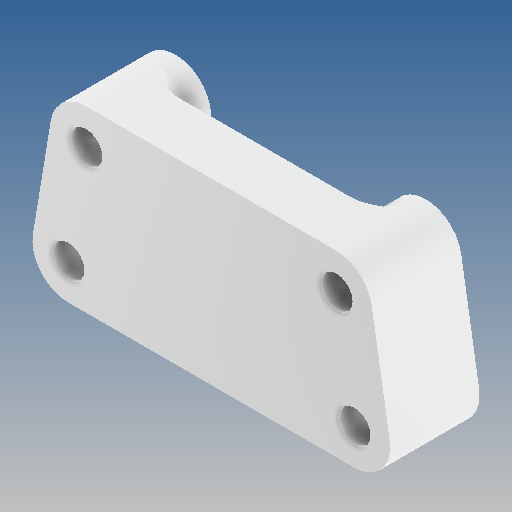
# Autodesk Inventor part: PWTR-0083
Saved by Autodesk Inventor 2021.1 (Build 251245000, 245)
## iProperties
Created: 2020-08-28
Part Number: PWTR-0083
Material: Aluminum 6061
Document SubType Name: Modeling
Designer: alid
Density: 2.7 g/cm^3
Appearance: Aluminum - Flat
Description: Handle Transfer Case Plate
Author: alid
Revision Number: A
Autodesk Inventor part; units mm, degrees
ref_plane "YZ Plane" through (0, 0, 0) normal (1, 0, 0) x (0, 1, 0)
ref_plane "XZ Plane" through (0, 0, 0) normal (0, 1, 0) x (-1, 0, 0)
ref_plane "XY Plane" through (0, 0, 0) normal (0, 0, 1) x (1, 0, 0)
sketch "Sketch1" plane through (0, 0, 0) normal (0, 1, 0) x (-1, 0, 0)
  line L0 (-40, -25) -> (40, -25)
  line L1 (35, 25) -> (-35, 25)
  line L2 (-49.863939, -13.35601) -> (-44.863939, 16.64399)
  line L3 (44.863939, 16.64399) -> (49.863939, -13.35601)
  circle A0 centre (-35, 15) radius 10
  circle A1 centre (-40, -15) radius 10
  circle A2 centre (35, 15) radius 10
  circle A3 centre (40, -15) radius 10
  line L4 (-35, 5) -> (35, 5)
  line L5 (-40, -5) -> (40, -5)
  line L6 (30.136061, -16.64399) -> (25.136061, 13.35601)
  line L7 (-25.136061, 13.35601) -> (-30.136061, -16.64399)
  point P0 (0, 0)
  point P1 (51.804604, -25)
  point P2 (0, 25)
  point P3 (0, -25)
  point P4 (0, -25)
  point P5 (-44.863939, 16.64399)
  dimension "d22" = 70
  dimension "d23" = 50
  dimension "d24" = 25
  dimension "d25" = 80
  dimension "d26" = 20
  constraints: 16 end point, 16 tangent, 15 point on circle, 4 centre point, 3 coincident, 3 equal radius, 3 midpoint, 3 vertical alignment, 2 point on line, 1 equal length, 1 horizontal, 1 parallel
  measures "d22" distance of L1.start L1.end
  measures "d23" distance between parallel lines of L0 L1
  measures "d24" distance from line of L0 point (0, 0)
  measures "d25" distance of L0.start L0.end
  measures "d26" diameter of A0
extrude "Extrusion1" add sketch "Sketch1" along normal blind 15
extrude "Extrusion2" add sketch "Sketch1" along normal blind 25 contours A1 | A3 | L2 A0 L4 L7 L5 A1 | A1 L5 L7 | L6 L5 A3 | A0 | L5 L6 L4 A2 L3 A3 | A0 L7 L4 | L6 A2 L4 | A2
fillet "Fillet1" radius 5 6 edges at (-27.6361, 15, -1.644) (-27.3698, 15, 21.4637) (-33.5363, 15, -22.6302) (27.6361, 15, -1.644) (33.5363, 15, -22.6302) (27.3698, 15, 21.4637)
hole "Hole2" at (-35, 0, 15) direction (0, 1, 0) diameter 9 end through all clearance for "Hex Head Cap Screw ISO 24017" size "M8" standard "ISO"
pattern_sketch "Sketch Driven Pattern1" of "Hole2" from (-35, 0, 15) copies at (-40, 0, -15) at (40, 0, -15) at (35, 0, 15)
equation "\"d24\" = 0.5 * d23"
body "Solid1"
